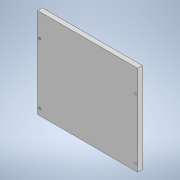
# Autodesk Inventor part: mávač_víčko
Saved by Autodesk Inventor 2022 (Build 260153000, 153)
## iProperties
Created: 2022-06-11
Part Number: mávač_víčko
Material: Generic
Document SubType Name: Modeling
Designer: Ruslana Zubareva
Density: 1 g/cm^3
Appearance: Default
Author: Ruslana Zubareva
Autodesk Inventor part; units mm, degrees
ref_plane "YZ Plane" through (0, 0, 0) normal (1, 0, 0) x (0, 1, 0)
ref_plane "XZ Plane" through (0, 0, 0) normal (0, 1, 0) x (-1, 0, 0)
ref_plane "XY Plane" through (0, 0, 0) normal (0, 0, 1) x (1, 0, 0)
sketch "Sketch1" plane through (0, 0, 0) normal (0, 0, 1) x (1, 0, 0)
  line L0 (0, 0) -> (150, 0)
  line L1 (150, 0) -> (150, -135)
  line L2 (150, -135) -> (0, -135)
  line L3 (0, -135) -> (0, 0)
  circle A0 centre (3.5, -35) radius 1.5
  line L4 (75, 0) -> (75, -135)
  circle A1 centre (146.5, -35) radius 1.5
  circle A2 centre (3.5, -125) radius 1.5
  circle A3 centre (146.5, -125) radius 1.5
  dimension "d0" = 150
  dimension "d1" = 135
  dimension "d2" = 3
  dimension "d3" = 3.5
  dimension "d4" = 35
  dimension "d5" = 3
  dimension "d6" = 3.5
  dimension "d7" = 90
  constraints: 10 end point, 4 centre point, 2 midpoint, 2 parallel, 2 symmetric about line, 1 horizontal, 1 perpendicular, 2 other
  measures "d0" distance of L1.end L2.end
  measures "d1" distance of L0.end L1.end
  measures "d2" diameter of A0
  measures "d3" distance from line of L3 A0.centre
  measures "d4" distance from line of L0 A0.centre
  measures "d5" diameter of A2
  measures "d6" distance from line of L3 A2.centre
  measures "d7" distance of A2.centre A0.centre
extrude "Extrusion1" add sketch "Sketch1" along normal blind 7
move faces "Move1" translate (0, -0.3, 0) faces at (100, 0, 2.3333)
move faces "Move2" translate (-0.3, 0, 0) faces at (150, -90.1, 2.3333)
move faces "Move3" translate (0, 0.3, 0) faces at (49.9, -135, 2.3333)
move faces "Move4" translate (0.3, 0, 0) faces at (0, -45.1, 2.3333)
body "Solid1"
